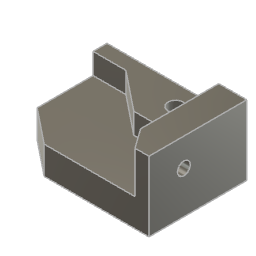
RoboconTask1 v0 (Autodesk Fusion 360 design; units mm, degrees)
Autodesk Fusion 360 part; units mm, degrees
note: some values were not read from the file. Chosen so that the rebuilt part matches the saved one: a direction.
sketch "Sketch1" plane through (0, 0, 0) normal (0, 1, 0) x (1, 0, 0)
  line L0 (-50, 50) -> (50, 50)
  line L1 (50, 50) -> (50, -20)
  line L2 (50, -20) -> (-25, -20)
  line L3 (-50, 0) -> (-50, 50)
  line L4 (-25, -20) -> (-50, 0)
  constraint horizontal L0
  constraint vertical L1
  constraint horizontal L2
  constraint vertical L3
extrude "Extrude1" add sketch "Sketch1" along normal blind 20
sketch "Sketch2" plane through (0, 20, 0) normal (0, 1, 0) x (-1, 0, 0)
  line L0 (25, 20) -> (-50, 20)
  line L1 (-50, 20) -> (-50, -50)
  line L2 (-50, -50) -> (50, -50)
  line L3 (50, -50) -> (50, 0)
  line L4 (50, 0) -> (25, 20)
  line L5 (-50, 20) -> (-50, -50)
  line L6 (25, 20) -> (-50, 20)
  line L7 (50, 0) -> (25, 20)
  line L8 (50, -50) -> (50, 0)
  line L9 (-50, -50) -> (50, -50)
  line L10 (50, -40) -> (26.5041, -40)
  line L11 (26.5041, -40) -> (-1.6201, -17.5006)
  line L12 (-1.6201, -17.5006) -> (-30, -17.5006)
  line L13 (-30, -17.5006) -> (-30, 5.9595)
  line L14 (-30, 5.9595) -> (-40, 20)
  circle A0 centre (-13.6491, -35.3724) radius 5.4442
  line L15 (-30, -17.5006) -> (-30, -50)
  constraint coincident L8 L10.start
  constraint perpendicular L8 L10
  constraint parallel L4 L11
  constraint horizontal L12
  constraint perpendicular L12 L13
  constraint coincident L6 L14.end
  constraint coincident L9 L15.end
  constraint perpendicular L9 L15
extrude "Extrude2" add sketch "Sketch2" along normal blind 15 contours L2 L3 L8 L9 L10 L11 L12 L15
extrude "Extrude3" add sketch "Sketch2" along normal blind 30 contours L0 L1 L2 L5 L6 L9 L13 L14 L15
sketch "Sketch3" plane through (30, 0, 0) normal (-1, 0, 0) x (0, 0, 1)
  line L0 (-50, 35) -> (-17.5006, 35)
  line L1 (-17.5006, 35) -> (-17.5006, 20)
  line L2 (-17.5006, 20) -> (5.9595, 20)
  line L3 (5.9595, 20) -> (5.9595, 50)
  line L4 (5.9595, 50) -> (-50, 50)
  line L5 (-50, 50) -> (-50, 35)
  circle A0 centre (-5, 30) radius 4.5807
extrude "Extrude4" cut sketch "Sketch3" against normal through all contours A0
